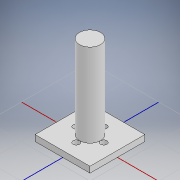
# Autodesk Inventor part: 000.001.015 - Стойка площадки высокая
Saved by Autodesk Inventor 2022 (Build 260153000, 153)
## iProperties
Created: 2023-06-09
Part Number: 000.001.015 - Стойка площадки высокая
Material: Типовые
Document SubType Name: Modeling
Designer: Иван Петров
Density: 1 g/cm^3
Appearance: По умолчанию
Author: Иван Петров
Autodesk Inventor part; units mm, degrees
ref_plane "YZ Plane" through (0, 0, 0) normal (1, 0, 0) x (0, 1, 0)
ref_plane "XZ Plane" through (0, 0, 0) normal (0, 1, 0) x (-1, 0, 0)
ref_plane "XY Plane" through (0, 0, 0) normal (0, 0, 1) x (1, 0, 0)
sketch "Эскиз1" plane through (0, 0, 0) normal (0, 1, 0) x (-1, 0, 0)
  line L0 (-16, 16) -> (16, 16)
  line L1 (16, 16) -> (16, -16)
  line L2 (16, -16) -> (-16, -16)
  line L3 (-16, -16) -> (-16, 16)
  line L4 (-16, 16) -> (16, -16) construction
  line L5 (16, 16) -> (-16, -16) construction
  point P0 (0, 0)
  dimension "d0" = 32
  dimension "d1" = 32
  constraints: 12 end point, 2 midpoint, 2 parallel, 1 horizontal, 1 perpendicular
  measures "d0" distance of L1.end L2.end
  measures "d1" distance of L0.end L1.end
extrude "Выдавливание1" add sketch "Эскиз1" along normal blind 3.5
sketch "Эскиз2" plane through (0, 3.5, 0) normal (0, 1, 0) x (1, 0, 0)
  circle A0 centre (0, 8) radius 1.85
  circle A1 centre (-5.6569, 5.6569) radius 1.85
  circle A2 centre (-8, 0) radius 1.85
  circle A3 centre (-5.6569, -5.6569) radius 1.85
  circle A4 centre (0, -8) radius 1.85
  circle A5 centre (5.6569, -5.6569) radius 1.85
  circle A6 centre (8, 0) radius 1.85
  circle A7 centre (5.6569, 5.6569) radius 1.85
  circle A8 centre (0, 0) radius 4
  circle A9 centre (0, 8) radius 1.85
  circle A10 centre (-5.6569, 5.6569) radius 1.85
  circle A11 centre (-8, 0) radius 1.85
  circle A12 centre (-5.6569, -5.6569) radius 1.85
  circle A13 centre (0, -8) radius 1.85
  circle A14 centre (5.6569, -5.6569) radius 1.85
  circle A15 centre (8, 0) radius 1.85
  circle A16 centre (5.6569, 5.6569) radius 1.85
  circle A17 centre (0, 0) radius 4
  circle A18 centre (0, 8) radius 1.85
  circle A19 centre (-5.6569, 5.6569) radius 1.85
  circle A20 centre (-8, 0) radius 1.85
  circle A21 centre (-5.6569, -5.6569) radius 1.85
  circle A22 centre (0, -8) radius 1.85
  circle A23 centre (5.6569, -5.6569) radius 1.85
  circle A24 centre (8, 0) radius 1.85
  circle A25 centre (5.6569, 5.6569) radius 1.85
  circle A26 centre (0, 0) radius 4
  point P0 (0, 0)
  point P1 (0, -16)
  point P2 (0, -16)
  point P3 (0, -16)
  constraints: 27 centre point
extrude "Выдавливание2" cut sketch "Эскиз2" against normal blind 3.5 contours A0 | A2 | A4 | A6
sketch "Эскиз3" plane through (0, 3.5, 0) normal (0, 1, 0) x (1, 0, 0)
  circle A0 centre (0, 0) radius 6.15
  circle A1 centre (-8, 0) radius 1.85 projected
  constraints: 1 centre point, 1 coincident, 1 tangent
extrude "Выдавливание3" add sketch "Эскиз3" along normal blind 48.5 contours A0
